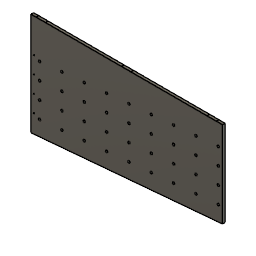
_PlywoodShelfBoard.d36e9c2d-b869-4dfb-9c43-cc4f85b06058 (Autodesk Fusion 360 design; units mm, degrees)
Autodesk Fusion 360 part; units mm, degrees
sketch "Sketch1" plane through (0, 0, 0) normal (0, 0, 1) x (1, 0, 0)
  line L0 (0, 0) -> (914.4, 0)
  line L1 (914.4, 0) -> (914.4, 600.8)
  line L2 (914.4, 600.8) -> (0, 600.8)
  line L3 (0, 600.8) -> (0, 0)
  dimension "d1" = 914.4
  dimension "d2" = 600.8
  constraint horizontal L0
  constraint vertical L1
  constraint horizontal L2
  constraint vertical L3
  constraint coincident L0.start L3.end
  measures "d1" distance of L0.start L0.end
  measures "d2" distance of L0.start L2.end
extrude "Extrude1" add sketch "Sketch1" along normal blind 6.35
sketch "Sketch4" plane through (0, 0, 6.35) normal (0, 0, 1) x (1, 0, 0)
  circle A0 centre (894.4, 150.8) radius 5.3675
  line L0 (0, 0) -> (800, 0)
  line L1 (914.4, 0) -> (914.4, 600.8)
  line L2 (0, 600.8) -> (0, 0)
  line L3 (0, 0) -> (914.4, 0)
  line L4 (914.4, 0) -> (914.4, 600.8)
  line L5 (914.4, 600.8) -> (0, 600.8)
  dimension "d6" = 10.735
  dimension "d8" = 150.8
  dimension "d38" = 20
  measures "d6" diameter of A0
  measures "d8" distance of A0.centre L0
  measures "d38" distance of A0.centre L1
extrude "Extrude2" cut sketch "Sketch4" against normal blind 35 contours A0
sketch "Sketch5" plane through (0, 0, 6.35) normal (0, 0, 1) x (1, 0, 0)
  circle A0 centre (894.4, 150.8) radius 5.3675
  line L0 (0, 600.8) -> (0, 0)
  line L1 (0, 0) -> (914.4, 0)
  line L2 (914.4, 0) -> (914.4, 600.8)
  line L3 (914.4, 600.8) -> (0, 600.8)
  line L4 (894.4, 150.8) -> (97.4442, 81.0754)
  line L5 (894.4, 150.8) -> (1694.4, 150.8) construction
  dimension "d11" = 175
  dimension "d12" = 800
  constraint horizontal L5
  constraint coincident A0.centre L4.start
  measures "d11" angle of L4 L5
  measures "d12" distance of A0.centre L4.end
pattern_linear "R-Pattern1" count 9 spacing 107 along (-0.996195, -0.087156, 0) count 4 spacing 80 along (0, 1, 0) of "Extrude2"
sketch "Sketch6" plane through (0, 0, 6.35) normal (0, 0, 1) x (1, 0, 0)
  circle A0 centre (41.6573, 316.1947) radius 5.3675
  circle A1 centre (148.2502, 325.5203) radius 5.3675
  circle A2 centre (254.843, 334.846) radius 5.3675
  circle A3 centre (361.4358, 344.1717) radius 5.3675
  circle A4 centre (468.0287, 353.4973) radius 5.3675
  circle A5 centre (574.6215, 362.823) radius 5.3675
  circle A6 centre (681.2143, 372.1487) radius 5.3675
  circle A7 centre (787.8072, 381.4743) radius 5.3675
  circle A8 centre (894.4, 390.8) radius 5.3675
  circle A9 centre (41.6573, 236.1947) radius 5.3675
  circle A10 centre (148.2502, 245.5203) radius 5.3675
  circle A11 centre (254.843, 254.846) radius 5.3675
  circle A12 centre (361.4358, 264.1717) radius 5.3675
  circle A13 centre (468.0287, 273.4973) radius 5.3675
  circle A14 centre (574.6215, 282.823) radius 5.3675
  circle A15 centre (681.2143, 292.1487) radius 5.3675
  circle A16 centre (787.8072, 301.4743) radius 5.3675
  circle A17 centre (894.4, 310.8) radius 5.3675
  circle A18 centre (41.6573, 156.1947) radius 5.3675
  circle A19 centre (148.2502, 165.5203) radius 5.3675
  circle A20 centre (254.843, 174.846) radius 5.3675
  circle A21 centre (361.4358, 184.1717) radius 5.3675
  circle A22 centre (468.0287, 193.4973) radius 5.3675
  circle A23 centre (574.6215, 202.823) radius 5.3675
  circle A24 centre (681.2143, 212.1487) radius 5.3675
  circle A25 centre (787.8072, 221.4743) radius 5.3675
  circle A26 centre (894.4, 230.8) radius 5.3675
  circle A27 centre (41.6573, 76.1947) radius 5.3675
  circle A28 centre (148.2502, 85.5203) radius 5.3675
  circle A29 centre (254.843, 94.846) radius 5.3675
  circle A30 centre (361.4358, 104.1717) radius 5.3675
  circle A31 centre (468.0287, 113.4973) radius 5.3675
  circle A32 centre (574.6215, 122.823) radius 5.3675
  circle A33 centre (681.2143, 132.1487) radius 5.3675
  circle A34 centre (787.8072, 141.4743) radius 5.3675
  circle A35 centre (894.4, 150.8) radius 5.3675
  line L0 (0, 600.8) -> (0, 0)
  line L1 (0, 0) -> (914.4, 0)
  line L2 (914.4, 0) -> (914.4, 600.8)
  line L3 (914.4, 600.8) -> (0, 600.8)
  line L4 (69.85, 567.0244) -> (69.85, 471.7744)
  line L5 (69.85, 471.7744) -> (25.4, 471.7744)
  line L6 (25.4, 471.7744) -> (25.4, 567.024)
  line L7 (25.4, 567.024) -> (69.85, 567.0244)
  line L8 (0, 600.8) -> (0, 0)
  line L9 (914.4, 600.8) -> (0, 600.8)
  line L10 (0, 0) -> (800, 0)
  dimension "d17" = 95.25
  dimension "d18" = 44.45
  dimension "d39" = 25.4
  dimension "d42" = 44.45
  dimension "d43" = 471.7744
  measures "d17" distance of L4.start L4.end
  measures "d18" distance of L4.start L6.end
  measures "d39" distance of L6 L8
  measures "d42" horizontal distance of L4.end L5.end
  measures "d43" distance of L5 L10
extrude "Extrude3" cut sketch "Sketch6" against normal blind 100 contours L4 L5 L6 L7
pattern_linear "R-Pattern2" count 3 spacing 407.5 along (1, 0, 0) of "Extrude3"
sketch "Sketch7" plane through (0, 0, 6.35) normal (0, 0, 1) x (1, 0, 0)
  line L0 (884.85, 471.7744) -> (840.4, 471.7744)
  line L1 (840.4, 471.7744) -> (840.4, 567.024)
  line L2 (840.4, 567.024) -> (884.85, 567.0244)
  line L3 (884.85, 567.0244) -> (884.85, 471.7744)
  line L4 (477.35, 471.7744) -> (432.9, 471.7744)
  line L5 (432.9, 471.7744) -> (432.9, 567.024)
  line L6 (432.9, 567.024) -> (477.35, 567.0244)
  line L7 (477.35, 567.0244) -> (477.35, 471.7744)
  line L8 (69.85, 471.7744) -> (25.4, 471.7744)
  line L9 (25.4, 471.7744) -> (25.4, 567.024)
  line L10 (25.4, 567.024) -> (69.85, 567.0244)
  line L11 (69.85, 567.0244) -> (69.85, 471.7744)
  circle A0 centre (41.6573, 316.1947) radius 5.3675
  circle A1 centre (148.2502, 325.5203) radius 5.3675
  circle A2 centre (254.843, 334.846) radius 5.3675
  circle A3 centre (361.4358, 344.1717) radius 5.3675
  circle A4 centre (468.0287, 353.4973) radius 5.3675
  circle A5 centre (574.6215, 362.823) radius 5.3675
  circle A6 centre (681.2143, 372.1487) radius 5.3675
  circle A7 centre (787.8072, 381.4743) radius 5.3675
  circle A8 centre (894.4, 390.8) radius 5.3675
  circle A9 centre (41.6573, 236.1947) radius 5.3675
  circle A10 centre (148.2502, 245.5203) radius 5.3675
  circle A11 centre (254.843, 254.846) radius 5.3675
  circle A12 centre (361.4358, 264.1717) radius 5.3675
  circle A13 centre (468.0287, 273.4973) radius 5.3675
  circle A14 centre (574.6215, 282.823) radius 5.3675
  circle A15 centre (681.2143, 292.1487) radius 5.3675
  circle A16 centre (787.8072, 301.4743) radius 5.3675
  circle A17 centre (894.4, 310.8) radius 5.3675
  circle A18 centre (41.6573, 156.1947) radius 5.3675
  circle A19 centre (148.2502, 165.5203) radius 5.3675
  circle A20 centre (254.843, 174.846) radius 5.3675
  circle A21 centre (361.4358, 184.1717) radius 5.3675
  circle A22 centre (468.0287, 193.4973) radius 5.3675
  circle A23 centre (574.6215, 202.823) radius 5.3675
  circle A24 centre (681.2143, 212.1487) radius 5.3675
  circle A25 centre (787.8072, 221.4743) radius 5.3675
  circle A26 centre (894.4, 230.8) radius 5.3675
  circle A27 centre (41.6573, 76.1947) radius 5.3675
  circle A28 centre (148.2502, 85.5203) radius 5.3675
  circle A29 centre (254.843, 94.846) radius 5.3675
  circle A30 centre (361.4358, 104.1717) radius 5.3675
  circle A31 centre (468.0287, 113.4973) radius 5.3675
  circle A32 centre (574.6215, 122.823) radius 5.3675
  circle A33 centre (681.2143, 132.1487) radius 5.3675
  circle A34 centre (787.8072, 141.4743) radius 5.3675
  circle A35 centre (894.4, 150.8) radius 5.3675
  line L12 (0, 600.8) -> (0, 0)
  line L13 (0, 0) -> (914.4, 0)
  line L14 (914.4, 0) -> (914.4, 600.8)
  line L15 (914.4, 600.8) -> (0, 600.8)
  line L16 (0, 0) -> (914.4, 79.9996)
  line L17 (0, 0) -> (803.0559, 0) construction
  line L18 (914.4, 79.9996) -> (914.4, 0)
  line L19 (914.4, 0) -> (0, 0)
  dimension "d25" = 5
  constraint horizontal L17
  constraint coincident L12.end L13.start
  constraint coincident L14 L16.end
  constraint coincident L13.end L14.start
  measures "d25" angle of L16 L17
extrude "Extrude4" cut sketch "Sketch7" against normal blind 150 contours L13 L14 L16 L18 L19
sketch "Sketch8" plane through (0, 0, 6.35) normal (0, 0, 1) x (1, 0, 0)
  line L0 (0, 0) -> (914.4, 79.9996)
  line L1 (914.4, 79.9996) -> (914.4, 600.8)
  line L2 (914.4, 600.8) -> (0, 600.8)
  line L3 (0, 600.8) -> (0, 0)
  circle A0 centre (894.4, 150.8) radius 5.3675
  circle A1 centre (787.8072, 141.4743) radius 5.3675
  circle A2 centre (681.2143, 132.1487) radius 5.3675
  circle A3 centre (574.6215, 122.823) radius 5.3675
  circle A4 centre (468.0287, 113.4973) radius 5.3675
  circle A5 centre (361.4358, 104.1717) radius 5.3675
  circle A6 centre (254.843, 94.846) radius 5.3675
  circle A7 centre (148.2502, 85.5203) radius 5.3675
  circle A8 centre (41.6573, 76.1947) radius 5.3675
  circle A9 centre (894.4, 230.8) radius 5.3675
  circle A10 centre (787.8072, 221.4743) radius 5.3675
  circle A11 centre (681.2143, 212.1487) radius 5.3675
  circle A12 centre (574.6215, 202.823) radius 5.3675
  circle A13 centre (468.0287, 193.4973) radius 5.3675
  circle A14 centre (361.4358, 184.1717) radius 5.3675
  circle A15 centre (254.843, 174.846) radius 5.3675
  circle A16 centre (148.2502, 165.5203) radius 5.3675
  circle A17 centre (41.6573, 156.1947) radius 5.3675
  circle A18 centre (894.4, 310.8) radius 5.3675
  circle A19 centre (787.8072, 301.4743) radius 5.3675
  circle A20 centre (681.2143, 292.1487) radius 5.3675
  circle A21 centre (574.6215, 282.823) radius 5.3675
  circle A22 centre (468.0287, 273.4973) radius 5.3675
  circle A23 centre (361.4358, 264.1717) radius 5.3675
  circle A24 centre (254.843, 254.846) radius 5.3675
  circle A25 centre (148.2502, 245.5203) radius 5.3675
  circle A26 centre (41.6573, 236.1947) radius 5.3675
  circle A27 centre (894.4, 390.8) radius 5.3675
  circle A28 centre (787.8072, 381.4743) radius 5.3675
  circle A29 centre (681.2143, 372.1487) radius 5.3675
  circle A30 centre (574.6215, 362.823) radius 5.3675
  circle A31 centre (468.0287, 353.4973) radius 5.3675
  circle A32 centre (361.4358, 344.1717) radius 5.3675
  circle A33 centre (254.843, 334.846) radius 5.3675
  circle A34 centre (148.2502, 325.5203) radius 5.3675
  circle A35 centre (41.6573, 316.1947) radius 5.3675
  line L4 (69.85, 471.7744) -> (25.4, 471.7744)
  line L5 (25.4, 471.7744) -> (25.4, 567.024)
  line L6 (25.4, 567.024) -> (69.85, 567.0244)
  line L7 (69.85, 567.0244) -> (69.85, 471.7744)
  line L8 (477.35, 471.7744) -> (432.9, 471.7744)
  line L9 (432.9, 471.7744) -> (432.9, 567.024)
  line L10 (432.9, 567.024) -> (477.35, 567.0244)
  line L11 (477.35, 567.0244) -> (477.35, 471.7744)
  line L12 (884.85, 471.7744) -> (840.4, 471.7744)
  line L13 (840.4, 471.7744) -> (840.4, 567.024)
  line L14 (840.4, 567.024) -> (884.85, 567.0244)
  line L15 (884.85, 567.0244) -> (884.85, 471.7744)
  circle A36 centre (15, 88.3) radius 2.25
  dimension "d28" = 4.5
  dimension "d29" = 88.3
  dimension "d30" = 15
  measures "d28" diameter of A36
  measures "d29" vertical distance of L0.start A36.centre
  measures "d30" distance of L3 A36.centre
extrude "Extrude5" cut sketch "Sketch8" against normal blind 35 contours A36
pattern_linear "R-Pattern3" count 4 spacing 80 along (0, 1, 0) of "Extrude5"
sketch "Sketch9" plane through (0, 0, 6.35) normal (0, 0, 1) x (1, 0, 0)
  circle A0 centre (15, 328.3) radius 2.25
  circle A1 centre (15, 248.3) radius 2.25
  circle A2 centre (15, 168.3) radius 2.25
  circle A3 centre (15, 88.3) radius 2.25
  line L0 (0, 0) -> (914.4, 79.9996)
  line L1 (914.4, 79.9996) -> (914.4, 600.8)
  line L2 (914.4, 600.8) -> (0, 600.8)
  line L3 (0, 600.8) -> (0, 0)
  circle A4 centre (894.4, 150.8) radius 5.3675
  circle A5 centre (787.8072, 141.4743) radius 5.3675
  circle A6 centre (681.2143, 132.1487) radius 5.3675
  circle A7 centre (574.6215, 122.823) radius 5.3675
  circle A8 centre (468.0287, 113.4973) radius 5.3675
  circle A9 centre (361.4358, 104.1717) radius 5.3675
  circle A10 centre (254.843, 94.846) radius 5.3675
  circle A11 centre (148.2502, 85.5203) radius 5.3675
  circle A12 centre (41.6573, 76.1947) radius 5.3675
  circle A13 centre (894.4, 230.8) radius 5.3675
  circle A14 centre (787.8072, 221.4743) radius 5.3675
  circle A15 centre (681.2143, 212.1487) radius 5.3675
  circle A16 centre (574.6215, 202.823) radius 5.3675
  circle A17 centre (468.0287, 193.4973) radius 5.3675
  circle A18 centre (361.4358, 184.1717) radius 5.3675
  circle A19 centre (254.843, 174.846) radius 5.3675
  circle A20 centre (148.2502, 165.5203) radius 5.3675
  circle A21 centre (41.6573, 156.1947) radius 5.3675
  circle A22 centre (894.4, 310.8) radius 5.3675
  circle A23 centre (787.8072, 301.4743) radius 5.3675
  circle A24 centre (681.2143, 292.1487) radius 5.3675
  circle A25 centre (574.6215, 282.823) radius 5.3675
  circle A26 centre (468.0287, 273.4973) radius 5.3675
  circle A27 centre (361.4358, 264.1717) radius 5.3675
  circle A28 centre (254.843, 254.846) radius 5.3675
  circle A29 centre (148.2502, 245.5203) radius 5.3675
  circle A30 centre (41.6573, 236.1947) radius 5.3675
  circle A31 centre (894.4, 390.8) radius 5.3675
  circle A32 centre (787.8072, 381.4743) radius 5.3675
  circle A33 centre (681.2143, 372.1487) radius 5.3675
  circle A34 centre (574.6215, 362.823) radius 5.3675
  circle A35 centre (468.0287, 353.4973) radius 5.3675
  circle A36 centre (361.4358, 344.1717) radius 5.3675
  circle A37 centre (254.843, 334.846) radius 5.3675
  circle A38 centre (148.2502, 325.5203) radius 5.3675
  circle A39 centre (41.6573, 316.1947) radius 5.3675
  line L4 (69.85, 471.7744) -> (25.4, 471.7744)
  line L5 (25.4, 471.7744) -> (25.4, 567.024)
  line L6 (25.4, 567.024) -> (69.85, 567.0244)
  line L7 (69.85, 567.0244) -> (69.85, 471.7744)
  line L8 (477.35, 471.7744) -> (432.9, 471.7744)
  line L9 (432.9, 471.7744) -> (432.9, 567.024)
  line L10 (432.9, 567.024) -> (477.35, 567.0244)
  line L11 (477.35, 567.0244) -> (477.35, 471.7744)
  line L12 (884.85, 471.7744) -> (840.4, 471.7744)
  line L13 (840.4, 471.7744) -> (840.4, 567.024)
  line L14 (840.4, 567.024) -> (884.85, 567.0244)
  line L15 (884.85, 567.0244) -> (884.85, 471.7744)
  line L16 (0, 0) -> (38.1, 0)
  line L17 (38.1, 0) -> (38.1, 50.8)
  line L18 (38.1, 50.8) -> (0, 50.8)
  line L19 (0, 50.8) -> (0, 0)
  line L20 (876.3, 79.9996) -> (876.3, 130.7996)
  line L21 (876.3, 130.7996) -> (914.4, 130.7996)
  line L22 (914.4, 130.7996) -> (914.4, 79.9996)
  line L23 (876.3, 79.9996) -> (876.3, 76.6663)
  line L24 (914.4, 79.9996) -> (876.3, 76.6663)
  dimension "d44" = 38.1
  dimension "d45" = 50.8
  dimension "d46" = 38.1
  dimension "d47" = 50.8
  constraint horizontal L16
  constraint vertical L17
  constraint horizontal L18
  constraint vertical L19
  constraint coincident L0.start L3.end
  constraint vertical L20
  constraint horizontal L21
  constraint vertical L22
  constraint coincident L0.end L1.start
  measures "d44" distance of L0.start L16.end
  measures "d45" distance of L0.start L18.end
  measures "d46" distance of L0.end L20.start
  measures "d47" distance of L0.end L21.end
extrude "Extrude6" cut sketch "Sketch9" against normal through all contours L0 L1 L20 L21 L22 L23 L24 | L0 L3 L17 L18 L19
sketch "Sketch10" plane through (0, 0, 6.35) normal (0, 0, 1) x (1, 0, 0)
  line L0 (884.85, 471.7744) -> (840.4, 471.7744)
  line L1 (840.4, 471.7744) -> (840.4, 567.024)
  line L2 (840.4, 567.024) -> (884.85, 567.0244)
  line L3 (884.85, 567.0244) -> (884.85, 471.7744)
  line L4 (477.35, 471.7744) -> (432.9, 471.7744)
  line L5 (432.9, 471.7744) -> (432.9, 567.024)
  line L6 (432.9, 567.024) -> (477.35, 567.0244)
  line L7 (477.35, 567.0244) -> (477.35, 471.7744)
  line L8 (69.85, 471.7744) -> (25.4, 471.7744)
  line L9 (25.4, 471.7744) -> (25.4, 567.024)
  line L10 (25.4, 567.024) -> (69.85, 567.0244)
  line L11 (69.85, 567.0244) -> (69.85, 471.7744)
  circle A0 centre (41.6573, 316.1947) radius 5.3675
  circle A1 centre (148.2502, 325.5203) radius 5.3675
  circle A2 centre (254.843, 334.846) radius 5.3675
  circle A3 centre (361.4358, 344.1717) radius 5.3675
  circle A4 centre (468.0287, 353.4973) radius 5.3675
  circle A5 centre (574.6215, 362.823) radius 5.3675
  circle A6 centre (681.2143, 372.1487) radius 5.3675
  circle A7 centre (787.8072, 381.4743) radius 5.3675
  circle A8 centre (894.4, 390.8) radius 5.3675
  circle A9 centre (41.6573, 236.1947) radius 5.3675
  circle A10 centre (148.2502, 245.5203) radius 5.3675
  circle A11 centre (254.843, 254.846) radius 5.3675
  circle A12 centre (361.4358, 264.1717) radius 5.3675
  circle A13 centre (468.0287, 273.4973) radius 5.3675
  circle A14 centre (574.6215, 282.823) radius 5.3675
  circle A15 centre (681.2143, 292.1487) radius 5.3675
  circle A16 centre (787.8072, 301.4743) radius 5.3675
  circle A17 centre (894.4, 310.8) radius 5.3675
  circle A18 centre (41.6573, 156.1947) radius 5.3675
  circle A19 centre (148.2502, 165.5203) radius 5.3675
  circle A20 centre (254.843, 174.846) radius 5.3675
  circle A21 centre (361.4358, 184.1717) radius 5.3675
  circle A22 centre (468.0287, 193.4973) radius 5.3675
  circle A23 centre (574.6215, 202.823) radius 5.3675
  circle A24 centre (681.2143, 212.1487) radius 5.3675
  circle A25 centre (787.8072, 221.4743) radius 5.3675
  circle A26 centre (894.4, 230.8) radius 5.3675
  circle A27 centre (41.6573, 76.1947) radius 5.3675
  circle A28 centre (148.2502, 85.5203) radius 5.3675
  circle A29 centre (254.843, 94.846) radius 5.3675
  circle A30 centre (361.4358, 104.1717) radius 5.3675
  circle A31 centre (468.0287, 113.4973) radius 5.3675
  circle A32 centre (574.6215, 122.823) radius 5.3675
  circle A33 centre (681.2143, 132.1487) radius 5.3675
  circle A34 centre (787.8072, 141.4743) radius 5.3675
  circle A35 centre (894.4, 150.8) radius 5.3675
  line L12 (876.3, 76.6663) -> (876.3, 130.7996)
  line L13 (876.3, 130.7996) -> (914.4, 130.7996)
  line L14 (914.4, 130.7996) -> (914.4, 600.8)
  line L15 (914.4, 600.8) -> (0, 600.8)
  line L16 (0, 600.8) -> (0, 50.8)
  line L17 (0, 50.8) -> (38.1, 50.8)
  line L18 (38.1, 50.8) -> (38.1, 3.3333)
  line L19 (38.1, 3.3333) -> (876.3, 76.6663)
  circle A36 centre (15, 88.3) radius 2.25
  circle A37 centre (15, 168.3) radius 2.25
  circle A38 centre (15, 248.3) radius 2.25
  circle A39 centre (15, 328.3) radius 2.25
  line L20 (0, 600.8) -> (914.4, 600.8)
  line L21 (914.4, 600.8) -> (914.4, 581.493)
  line L22 (0, 581.493) -> (0, 600.8)
  line L23 (0, 573.5444) -> (137.1702, 573.5444)
  line L24 (525.4366, 574.2351) -> (572.2435, 574.2351)
  line L25 (914.4, 600.8) -> (-15.3198, 600.8)
  line L26 (-15.3198, 600.8) -> (-15.3198, 592.064)
  line L27 (-15.3198, 592.064) -> (914.4, 592.064)
  line L28 (914.4, 592.064) -> (914.4, 600.8)
  dimension "d49" = 0.001
  dimension "d50" = 8.736
  constraint horizontal L20
  constraint vertical L21
  constraint vertical L22
  constraint coincident L15.end L16.start
  constraint coincident L16 L23.start
  constraint horizontal L25
  constraint vertical L26
  constraint horizontal L27
  constraint vertical L28
  constraint coincident L14.end L15.start
  measures "d49" angle of L6 L24
  measures "d50" distance of L14.end L27.end
extrude "Extrude7" cut sketch "Sketch10" against normal blind 175 contours L14 L15 L16 L20 L21 L22 L25 L27 L28
extrude "Extrude8" add 1 faces at (252.531, 491.4207, 6.35) along direction (0, 0, 1) blind 6.35
sketch "Sketch11" plane through (0, 0, 12.7) normal (0, 0, 1) x (1, 0, 0)
  circle A0 centre (15, 328.3) radius 2.25
  circle A1 centre (15, 248.3) radius 2.25
  circle A2 centre (15, 168.3) radius 2.25
  circle A3 centre (15, 88.3) radius 2.25
  line L0 (914.4, 592.064) -> (0, 592.064)
  line L1 (0, 592.064) -> (0, 50.8)
  line L2 (0, 50.8) -> (38.1, 50.8)
  line L3 (38.1, 50.8) -> (38.1, 3.3333)
  line L4 (38.1, 3.3333) -> (876.3, 76.6663)
  line L5 (876.3, 76.6663) -> (876.3, 130.7996)
  line L6 (876.3, 130.7996) -> (914.4, 130.7996)
  line L7 (914.4, 130.7996) -> (914.4, 592.064)
  circle A4 centre (894.4, 150.8) radius 5.3675
  circle A5 centre (787.8072, 141.4743) radius 5.3675
  circle A6 centre (681.2143, 132.1487) radius 5.3675
  circle A7 centre (574.6215, 122.823) radius 5.3675
  circle A8 centre (468.0287, 113.4973) radius 5.3675
  circle A9 centre (361.4358, 104.1717) radius 5.3675
  circle A10 centre (254.843, 94.846) radius 5.3675
  circle A11 centre (148.2502, 85.5203) radius 5.3675
  circle A12 centre (41.6573, 76.1947) radius 5.3675
  circle A13 centre (894.4, 230.8) radius 5.3675
  circle A14 centre (787.8072, 221.4743) radius 5.3675
  circle A15 centre (681.2143, 212.1487) radius 5.3675
  circle A16 centre (574.6215, 202.823) radius 5.3675
  circle A17 centre (468.0287, 193.4973) radius 5.3675
  circle A18 centre (361.4358, 184.1717) radius 5.3675
  circle A19 centre (254.843, 174.846) radius 5.3675
  circle A20 centre (148.2502, 165.5203) radius 5.3675
  circle A21 centre (41.6573, 156.1947) radius 5.3675
  circle A22 centre (894.4, 310.8) radius 5.3675
  circle A23 centre (787.8072, 301.4743) radius 5.3675
  circle A24 centre (681.2143, 292.1487) radius 5.3675
  circle A25 centre (574.6215, 282.823) radius 5.3675
  circle A26 centre (468.0287, 273.4973) radius 5.3675
  circle A27 centre (361.4358, 264.1717) radius 5.3675
  circle A28 centre (254.843, 254.846) radius 5.3675
  circle A29 centre (148.2502, 245.5203) radius 5.3675
  circle A30 centre (41.6573, 236.1947) radius 5.3675
  circle A31 centre (894.4, 390.8) radius 5.3675
  circle A32 centre (787.8072, 381.4743) radius 5.3675
  circle A33 centre (681.2143, 372.1487) radius 5.3675
  circle A34 centre (574.6215, 362.823) radius 5.3675
  circle A35 centre (468.0287, 353.4973) radius 5.3675
  circle A36 centre (361.4358, 344.1717) radius 5.3675
  circle A37 centre (254.843, 334.846) radius 5.3675
  circle A38 centre (148.2502, 325.5203) radius 5.3675
  circle A39 centre (41.6573, 316.1947) radius 5.3675
  line L8 (69.85, 471.7744) -> (25.4, 471.7744)
  line L9 (25.4, 471.7744) -> (25.4, 567.024)
  line L10 (25.4, 567.024) -> (69.85, 567.0244)
  line L11 (69.85, 567.0244) -> (69.85, 471.7744)
  line L12 (477.35, 471.7744) -> (432.9, 471.7744)
  line L13 (432.9, 471.7744) -> (432.9, 567.024)
  line L14 (432.9, 567.024) -> (477.35, 567.0244)
  line L15 (477.35, 567.0244) -> (477.35, 471.7744)
  line L16 (884.85, 471.7744) -> (840.4, 471.7744)
  line L17 (840.4, 471.7744) -> (840.4, 567.024)
  line L18 (840.4, 567.024) -> (884.85, 567.0244)
  line L19 (884.85, 567.0244) -> (884.85, 471.7744)
  line L20 (0, 592.064) -> (914.4, 592.064)
  line L21 (914.4, 592.064) -> (914.4, 490.464)
  line L22 (914.4, 490.464) -> (0, 490.464)
  line L23 (0, 490.464) -> (0, 592.064)
  dimension "d55" = 101.6
  constraint horizontal L20
  constraint vertical L21
  constraint horizontal L22
  constraint vertical L23
  constraint coincident L7 L21.end
  constraint coincident L0.end L1.start
  measures "d55" distance of L0.end L22.end
extrude "Extrude9" cut sketch "Sketch11" against normal through all contours L0 L1 L7 L9 L10 L11 L13 L14 L15 L17 L18 L19 L20 L21 L22 L23
move_face "OffsetFaces1" offset 18.69 3 faces at (855.2167, 471.7744, 8.4667) (462.5333, 471.7744, 8.4667) (40.2167, 471.7744, 8.4667)
convert_to_sheet_metal "ConvertToSheetMetal1"
delete_face "DeleteFace1" 2 faces at (889, 130.7996, 4.2333) (876.3, 94.7108, 8.4667)
delete_face "DeleteFace2" 2 faces at (25.4, 50.8, 4.2333) (38.1, 19.1555, 4.2333)
equation "d2 = 550 mm + 2 in"
equation "d8 = 100 mm + 2 in"
equation "d29 = 37.5 mm + 2 in"
equation "d43 = 420.9744283331 mm + 2 in"
